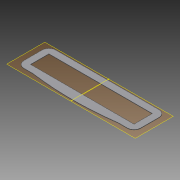
# Autodesk Inventor part: frontprofile
Saved by Autodesk Inventor 2014 SP1 (Build 180222100, 222)
## iProperties
Created: 2014-04-05
Part Number: frontprofile
Material: Generic
Document SubType Name: Modeling
Designer: Tyler
Density: 1 g/cm^3
Appearance: Default
Author: Tyler
Autodesk Inventor part; units mm, degrees
ref_plane "XZ Plane" through (0, 0, 0) normal (0, 1, 0) x (-1, 0, 0)
sketch "Sketch1" plane through (0, 0, 0) normal (0, 0, 1) x (1, 0, 0)
  line L0 (-62, 19) -> (62, 19)
  line L1 (70, 11) -> (70, -11)
  line L2 (62, -19) -> (-62, -19)
  line L3 (-70, -11) -> (-70, 11)
  arc A0 (70, 11) -> (62, 19) centre (62, 11) ccw
  arc A1 (62, -19) -> (70, -11) centre (62, -11) ccw
  arc A2 (-70, -11) -> (-62, -19) centre (-62, -11) ccw
  arc A3 (-62, 19) -> (-70, 11) centre (-62, 11) ccw
  point P0 (0, 0)
  dimension "d0" = 19
  dimension "d1" = 38
  dimension "d2" = 140
  dimension "d3" = 70
  dimension "d4" = 8
  dimension "d5" = 8
  constraints: 8 end point, 8 point on circle, 8 tangent, 4 centre point, 2 equal radius, 2 parallel, 1 horizontal, 1 perpendicular
  measures "d0" distance from line of point (0, 0) L0
  measures "d1" distance between parallel lines of L2 L0
  measures "d2" distance between parallel lines of L1 L3
  measures "d3" distance from line of L3 point (0, 0)
  measures "d4" radius of A0
  measures "d5" radius of A1
extrude "Extrusion1" add sketch "Sketch1" along normal blind 0.5
sketch "Sketch2" plane through (0, 0, 0) normal (0, 0, 1) x (1, 0, 0)
  arc A0 (-49.9899, -19.1353) -> (-52, -19) centre (-52, -34) ccw
  arc A1 (52, -19) -> (49.9899, -19.1353) centre (52, -34) ccw
  line L0 (52, -17) -> (52, -19)
  line L1 (70, -11) -> (70, 11) projected
  line L2 (-70, 11) -> (-70, -11) projected
  line L3 (-62, -19) -> (62, -19) projected
  line L4 (-52, -34) -> (-52, -17)
  line L5 (-52, -17) -> (52, -17)
  line L6 (52, -17) -> (52, -19)
  arc A2 (-49.9899, -19.1353) -> (49.9899, -19.1353) centre (0, 350.5357) ccw
  dimension "d24" = 30
  dimension "d25" = 30
  dimension "d26" = 18
  dimension "d27" = 15
  dimension "d28" = 15
  dimension "d30" = 2
  dimension "d31" = 18
  dimension "d32" = 5.5
  constraints: 8 end point, 6 point on circle, 3 centre point, 2 perpendicular, 2 point on line, 2 tangent, 1 parallel
  measures "d24" diameter of A1
  measures "d25" diameter of A0
  measures "d26" distance from line of L2 L4.start
  measures "d27" distance from line of L3 L4.start
  measures "d28" distance from line of L3 A1.centre
  measures "d30" distance between parallel lines of L3 L5
  measures "d31" distance from line of L1 A1.centre
  measures "d32" distance edge to line of A2 L5
extrude "Extrusion2" add sketch "Sketch2" along normal blind 0.5
sketch "Sketch3" plane through (0, 0, 0) normal (0, 0, 1) x (1, 0, 0)
  arc A0 (62, -19) -> (70, -11) centre (62, -11) ccw
  arc A1 (-62, 19) -> (-70, 11) centre (-62, 11) ccw
  line L0 (-62, 11) -> (62, 11)
  line L1 (62, 11) -> (62, -11)
  line L2 (62, -11) -> (-62, -11)
  line L3 (-62, -11) -> (-62, 11)
  point P0 (0, 0)
  constraints: 8 end point, 4 point on circle, 2 centre point, 2 parallel, 1 horizontal, 1 perpendicular
extrude "Extrusion3" cut sketch "Sketch3" along normal through all both and the other way through all
equation "\"d0\" = 0.5 * d1"
equation "\"d3\" = 0.5 * d2"
body "Solid1"
